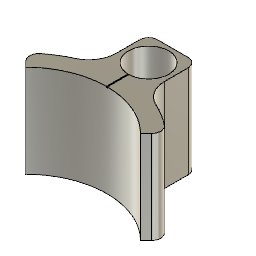
AvionicsTubeAttachment (Autodesk Fusion 360 design; units mm, degrees)
Autodesk Fusion 360 part; units mm, degrees
sketch "Sketch1" plane through (0, 0, 0) normal (0, 0, 1) x (1, 0, 0)
  circle A0 centre (0, 0) radius 44.45
  arc A1 (38.1661, 38.1661) -> (-38.1661, 38.1661) centre (0, 0) ccw
  line L0 (0, 0) -> (38.1661, 38.1661) construction
  line L1 (0, 0) -> (-38.1661, 38.1661) construction
  line L2 (-38.1661, 38.1661) -> (-31.4309, 31.4309) construction
  line L3 (-38.1661, 38.1661) -> (-31.4309, 31.4309)
  line L4 (31.4309, 31.4309) -> (38.1661, 38.1661)
  line L5 (0, 0) -> (0, 53.975) construction
  line L6 (0, 53.975) -> (-31.4309, 31.4309) construction
  line L7 (0, 53.975) -> (31.4309, 31.4309) construction
  line L8 (-13.335, 80.645) -> (13.335, 80.645)
  line L9 (13.335, 80.645) -> (13.335, 53.975)
  line L10 (13.335, 53.975) -> (-13.335, 53.975) construction
  line L11 (-13.335, 53.975) -> (-13.335, 80.645)
  line L12 (-13.335, 53.975) -> (-13.335, 52.3018)
  line L13 (13.335, 53.975) -> (13.335, 52.3018)
  line L14 (-13.335, 67.31) -> (13.335, 67.31) construction
  circle A2 centre (0, 67.31) radius 11.049
  point P0 (-31.4309, 31.4309)
  point P1 (-13.335, 52.3018)
  point P2 (13.335, 52.3018)
  point P3 (-13.335, 67.31)
  point P4 (13.335, 67.31)
  dimension "d1" = 88.9
  dimension "d2" = 90
  dimension "d3" = 9.525
  dimension "d6" = 26.67
  dimension "d7" = 26.67
  dimension "d8" = 22.098
  constraint coincident A0.centre A1.centre
  constraint coincident A0 P0
  constraint coincident L1 P0
  constraint coincident P0 L2.end
  constraint coincident A0 L4.start
  constraint coincident L0 L4.start
  constraint vertical L5
  constraint equal L6 L7
  constraint midpoint A1 L5.end
  constraint horizontal L8
  constraint vertical L9
  constraint horizontal L10
  constraint vertical L11
  constraint midpoint L5.end L10
  constraint coincident A1 P1
  constraint perpendicular L10 L12
  constraint coincident A1 P2
  constraint perpendicular L10 L13
  constraint coincident P1 L12.end
  constraint coincident P2 L13.end
  constraint coincident L11 P3
  constraint midpoint L11 P3
  constraint midpoint L9 P4
  constraint coincident P3 L14.start
  constraint coincident P4 L14.end
  constraint midpoint L14 A2.centre
  measures "d1" diameter of A0
  measures "d2" angle of L0 L1
  measures "d3" distance of A1.end P0
  measures "d6" distance of L8.start L8.end
  measures "d7" distance of L8.end L9.end
  measures "d8" diameter of A2
extrude "Extrude2" add sketch "Sketch1" along normal blind 50.8 contours A0 A1 L3 L4 | A1 L8 L9 L11 L12 L13
fillet "Fillet1" radius 5 2 edges at (-38.1661, 38.1661, 25.4) (38.1661, 38.1661, 25.4)
fillet "Fillet2" radius 15 2 edges at (-13.335, 52.3018, 25.4) (13.335, 52.3018, 25.4)
fillet "Fillet3" radius 5 2 edges at (-13.335, 80.645, 25.4) (13.335, 80.645, 25.4)
sketch "Sketch4" plane through (0, 80.645, 0) normal (0, 1, 0) x (-1, 0, 0)
  line L0 (-8.335, 50.8) -> (-8.335, 0)
  line L1 (-8.335, 0) -> (8.335, 0)
  line L2 (8.335, 0) -> (8.335, 50.8)
  line L3 (8.335, 50.8) -> (-8.335, 50.8)
  line L4 (0, 0) -> (0, 16.9333) construction
  line L5 (0, 16.9333) -> (0, 33.8667) construction
  line L6 (0, 33.8667) -> (0, 50.8) construction
  circle A0 centre (0, 16.9333) radius 1.778
  circle A1 centre (0, 33.8667) radius 1.778
  dimension "d17" = 3.556
  dimension "d18" = 3.556
  constraint coincident L4.start origin
  constraint perpendicular L1 L4
  constraint parallel L4 L5
  constraint midpoint L3 L6.end
  constraint equal L5 L6
  constraint equal L4 L5
  constraint coincident L4.end L5.start
  constraint coincident L5.end L6.start
  measures "d17" diameter of A0
  measures "d18" diameter of A1
extrude "Extrude3" cut sketch "Sketch4" along normal up to surface contours A0 | A1 end surface at (10.9941, 66.2099, 33.8667)
sketch "Sketch6" plane through (0, 0, 50.8) normal (0, 0, 1) x (-1, 0, 0)
  arc A0 (-13.335, -75.645) -> (-8.335, -80.645) centre (-8.335, -75.645) ccw
  line L0 (-8.335, -80.645) -> (8.335, -80.645)
  arc A1 (8.335, -80.645) -> (13.335, -75.645) centre (8.335, -75.645) ccw
  line L1 (13.335, -75.645) -> (13.335, -62.8862)
  arc A2 (22.173, -49.2104) -> (13.335, -62.8862) centre (28.335, -62.8862) ccw
  arc A3 (22.173, -49.2104) -> (34.0702, -41.8632) centre (0, 0) ccw
  arc A4 (34.0702, -41.8632) -> (34.4496, -34.4496) centre (30.9141, -37.9851) ccw
  line L2 (34.4496, -34.4496) -> (31.4309, -31.4309)
  arc A5 (-31.4309, -31.4309) -> (31.4309, -31.4309) centre (0, 0) ccw
  line L3 (-31.4309, -31.4309) -> (-34.4496, -34.4496)
  arc A6 (-34.4496, -34.4496) -> (-34.0702, -41.8632) centre (-30.9141, -37.9851) ccw
  arc A7 (-34.0702, -41.8632) -> (-22.173, -49.2104) centre (0, 0) ccw
  arc A8 (-13.335, -62.8862) -> (-22.173, -49.2104) centre (-28.335, -62.8862) ccw
  line L4 (-13.335, -62.8862) -> (-13.335, -75.645)
  circle A9 centre (0, -67.31) radius 11.049
  line L5 (0, -56.261) -> (0, -44.45)
  circle A10 centre (0, -67.31) radius 11.049
  circle A11 centre (0, 0) radius 44.45
  line L6 (0.25, -56.261) -> (-0.25, -56.261)
  line L7 (-0.25, -56.261) -> (-0.25, -44.45)
  line L8 (-0.25, -44.45) -> (0.25, -44.45)
  line L9 (0.25, -44.45) -> (0.25, -56.261)
  line L10 (0, 0) -> (0, -53.975)
  dimension "d22" = 0.5
  constraint vertical L5
  constraint coincident L5.start A10
  constraint coincident L5.end A11
  constraint horizontal L6
  constraint vertical L7
  constraint horizontal L8
  constraint vertical L9
  constraint midpoint L5.start L6
  constraint midpoint L5.end L8
  constraint collinear L5 L10
  measures "d22" distance of L6.start L6.end
extrude "Extrude4" cut sketch "Sketch6" against normal blind 0.5 contours L5 L6 L8 L9 L10 | L5 L6 L7 L8 L10
